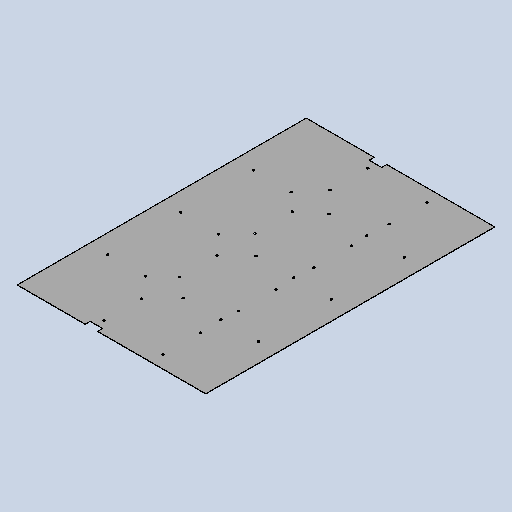
# Autodesk Inventor part: GnG L.3 floor sheet
Saved by Autodesk Inventor 2025.3 (Build 293356030, 356C)
## iProperties
Created: 2025-10-28
Part Number: GnG L.3 floor sheet
Material: Stainless Steel
Document SubType Name: Sheet Metal
Designer: admin
Mass: 82475.6 g
Surface Area: 69006.7 cm^2
Volume: 10309.4 cm^3
Density: 8 g/cm^3
Sheet Metal Rule: AISI304 3mm Die 32
Sheet Metal Width: 1500,000 mm
Sheet Metal Length: 2300,000 mm
Sheet Metal Area: 3450000,000 mm^2
Appearance: Default
Stock Number: L 3
Flat Pattern Width: 150 cm
Flat Pattern Length: 230 cm
Flat Pattern Area: 34500 cm^2
Author: admin
Autodesk Inventor part; units mm, degrees
ref_plane "YZ Plane" through (0, 0, 0) normal (1, 0, 0) x (0, 1, 0)
ref_plane "XZ Plane" through (0, 0, 0) normal (0, 1, 0) x (-1, 0, 0)
ref_plane "XY Plane" through (0, 0, 0) normal (0, 0, 1) x (1, 0, 0)
sketch "Sketch1" plane through (0, 0, 0) normal (0, 0, 1) x (1, 0, 0)
  line L0 (0, 0) -> (-1500, 0)
  line L1 (-1500, 0) -> (-1500, -2300)
  line L2 (-1500, -2300) -> (0, -2300)
  line L3 (0, -2300) -> (0, 0)
  line L4 (0, 0) -> (-40, 0)
  line L5 (-40, 0) -> (-40, -40)
  line L6 (-40, -40) -> (0, -40)
  line L7 (0, -40) -> (0, 0)
  line L8 (0, -2300) -> (-40, -2300)
  line L9 (-40, -2300) -> (-40, -2260)
  line L10 (-40, -2260) -> (0, -2260)
  line L11 (0, -2260) -> (0, -2300)
  line L12 (-1500, 0) -> (-1460, 0)
  line L13 (-1460, 0) -> (-1460, -40)
  line L14 (-1460, -40) -> (-1500, -40)
  line L15 (-1500, -40) -> (-1500, 0)
  line L16 (-1500, -2300) -> (-1460, -2300)
  line L17 (-1460, -2300) -> (-1460, -2260)
  line L18 (-1460, -2260) -> (-1500, -2260)
  line L19 (-1500, -2260) -> (-1500, -2300)
  line L20 (-960, -2300) -> (-860, -2300)
  line L21 (-860, -2300) -> (-860, -2260)
  line L22 (-860, -2260) -> (-960, -2260)
  line L23 (-960, -2260) -> (-960, -2300)
  line L24 (-960, 0) -> (-860, 0)
  line L25 (-860, 0) -> (-860, -40)
  line L26 (-860, -40) -> (-960, -40)
  line L27 (-960, -40) -> (-960, 0)
  point P0 (0, -40)
  point P1 (-40, 0)
  point P2 (0, -2260)
  point P3 (-860, 0)
  dimension "d22" = 1500
  dimension "d23" = 2300
  dimension "d24" = 40
  dimension "d25" = 40
  dimension "d28" = 100
  dimension "d29" = 820
  measures "d22" distance of L2.end L1.end
  measures "d23" distance of L1.end L0.end
  measures "d24" distance of L6.end L5.end
  measures "d25" distance of L5.end L4.end
  measures "d28" distance of L25.end L26.end
  measures "d29" distance between parallel lines of L5 L25
extrude "Plate1" add sketch "Sketch1" along normal blind 3 contours L3 L6 L5 L0 | L5 L6 L3 L10 L9 L2 L21 L22 L23 L17 L18 L1 L14 L13 L0 L27 L26 L25 | L3 L2 L9 L10 | L13 L14 L1 L0 | L18 L17 L2 L1
sketch "Sketch6" plane through (0, 0, 3) normal (0, 0, 1) x (1, 0, 0)
  line L0 (-1395, 0) -> (-1390, 0)
  line L1 (-1375, -2) -> (-1375, 0)
  line L2 (-1375, 0) -> (-1370, 0)
  line L3 (-1370, 0) -> (-1370, -2)
  line L4 (-1370, 0) -> (-1365, 0) construction
  line L5 (-1365, 0) -> (-1363.3887, -1.629)
  arc A0 (-1363.3887, -1.629) -> (-1361.6113, -1.629) centre (-1362.5, -0.75) ccw
  line L6 (-1365, 0) -> (-1360, 0)
  line L7 (-1360, 0) -> (-1355, 0) construction
  line L8 (-1355, -2) -> (-1355, 0)
  line L9 (-1350, -2) -> (-1355, -2)
  line L10 (-1350, 0) -> (-1350, -2)
  line L11 (-1355, 0) -> (-1350, 0)
  line L12 (-1350, -1) -> (-1345, -1) construction
  line L13 (-1361.6113, -1.629) -> (-1360, 0)
  line L14 (-1390, 0) -> (-1390, -2)
  line L15 (-1390, -2) -> (-1395, -2)
  line L16 (-1395, -2) -> (-1395, 0)
  line L17 (-1370, -2) -> (-1375, -2)
  line L18 (-1380, 0) -> (-1380, -2)
  line L19 (-1380, -2) -> (-1385, -2)
  line L20 (-1385, -2) -> (-1385, 0)
  line L21 (-1385, 0) -> (-1380, 0)
  line L22 (-1380, -1) -> (-1375, -1) construction
  line L23 (-1390, -1) -> (-1385, -1) construction
  line L24 (-1345, -2) -> (-1345, 0)
  line L25 (-1340, 0) -> (-1340, -2)
  line L26 (-1340, -2) -> (-1345, -2)
  line L27 (-1345, 0) -> (-1340, 0)
  line L28 (-1340, -1) -> (-1335, -1) construction
  line L29 (-1335, -2) -> (-1335, 0)
  line L30 (-1335, 0) -> (-1330, 0)
  line L31 (-1330, -2) -> (-1335, -2)
  arc A1 (-1402.5, 0) -> (-1397.5, 0) centre (-1400, 0) ccw
  line L32 (-1330, 0) -> (-1330, -2)
  line L33 (-1500, 0) -> (-960, 0) projected
  line L34 (-1500, -2300) -> (-1500, 0) projected
  point P0 (0, 0)
  point P1 (-1362.5, 0)
  dimension "d38" = 5
  dimension "d39" = 2
  dimension "d40" = 1.25
  dimension "d41" = 5
  dimension "d42" = 5
  dimension "d43" = 2
  dimension "d44" = 5
  dimension "d45" = 5
  dimension "d46" = 100
  constraints: 66 end point, 12 parallel, 11 horizontal, 10 equal length, 9 midpoint, 6 perpendicular, 5 collinear, 4 point on circle, 4 point on line, 3 tangent, 2 centre point, 1 vertical alignment
  measures "d38" distance of L14.end L16.start
  measures "d39" distance of L16.start L0.start
  measures "d40" radius of A0
  measures "d41" distance of L5.start L6.end
  measures "d42" distance of L10.end L8.start
  measures "d43" distance of L8.start L7.end
  measures "d44" diameter of A1
  measures "d45" distance of A1.centre L0.start
  measures "d46" distance from line of L34 A1.centre
extrude "Cut1" cut sketch "Sketch6" against normal blind 3 contours L2 L3 L17 L1 | L21 L18 L19 L20 | L0 L14 L15 L16 | A1 L33
sketch "Sketch7" plane through (0, 0, 0) normal (0, 0, -1) x (-1, 0, 0)
  line L0 (1375, 0) -> (1375, -2) construction
  line L1 (1375, -2) -> (1370, -2) construction
  line L2 (1370, -2) -> (1370, 0) construction
  line L3 (960, 0) -> (1370, 0) construction
  line L4 (960, -40) -> (960, 0) construction
  line L5 (860, -40) -> (960, -40) construction
  line L6 (860, 0) -> (860, -40) construction
  line L7 (0, 0) -> (860, 0) construction
  line L8 (0, -2300) -> (0, 0) construction
  line L9 (860, -2300) -> (0, -2300) construction
  line L10 (860, -2260) -> (860, -2300) construction
  line L11 (960, -2260) -> (860, -2260) construction
  line L12 (960, -2300) -> (960, -2260) construction
  line L13 (1500, -2300) -> (960, -2300) construction
  line L14 (1500, 0) -> (1500, -2300) construction
  line L15 (1402.5, 0) -> (1500, 0) construction
  arc A0 (1397.5, 0) -> (1402.5, 0) centre (1400, 0) ccw construction
  line L16 (1395, 0) -> (1397.5, 0) construction
  line L17 (1395, 0) -> (1395, -2) construction
  line L18 (1395, -2) -> (1390, -2) construction
  line L19 (1390, -2) -> (1390, 0) construction
  line L20 (1385, 0) -> (1390, 0) construction
  line L21 (1385, 0) -> (1385, -2) construction
  line L22 (1385, -2) -> (1380, -2) construction
  line L23 (1380, -2) -> (1380, 0) construction
  line L24 (1375, 0) -> (1380, 0) construction
  line L25 (440, 0) -> (440, -2300) construction
  line L26 (910, -2260) -> (910, -40) construction
  line L27 (1500, -570) -> (0, -570) construction
  line L28 (1500, -1150) -> (0, -1150) construction
  line L29 (1500, -1730) -> (0, -1730) construction
  circle A1 centre (440, -2200) radius 7.5
  circle A2 centre (910, -2200) radius 7.5
  circle A3 centre (1350, -570) radius 7.5
  circle A4 centre (1350, -1150) radius 7.5
  circle A5 centre (1350, -1730) radius 7.5
  circle A6 centre (910, -1900) radius 7.5
  circle A7 centre (440, -1900) radius 7.5
  circle A8 centre (910, -1600) radius 7.5
  circle A9 centre (440, -1600) radius 7.5
  circle A10 centre (910, -1300) radius 7.5
  circle A11 centre (440, -1300) radius 7.5
  circle A12 centre (910, -1000) radius 7.5
  circle A13 centre (440, -1000) radius 7.5
  circle A14 centre (910, -700) radius 7.5
  circle A15 centre (440, -700) radius 7.5
  circle A16 centre (910, -400) radius 7.5
  circle A17 centre (440, -400) radius 7.5
  circle A18 centre (910, -100) radius 7.5
  circle A19 centre (440, -100) radius 7.5
  circle A20 centre (910, 200) radius 7.5
  circle A21 centre (440, 200) radius 7.5
  circle A22 centre (910, 500) radius 7.5
  circle A23 centre (440, 500) radius 7.5
  circle A24 centre (910, 800) radius 7.5
  circle A25 centre (440, 800) radius 7.5
  circle A26 centre (1050, -1730) radius 7.5
  circle A27 centre (1050, -570) radius 7.5
  circle A28 centre (1050, -1150) radius 7.5
  circle A29 centre (750, -1730) radius 7.5
  circle A30 centre (750, -570) radius 7.5
  circle A31 centre (750, -1150) radius 7.5
  circle A32 centre (450, -1730) radius 7.5
  circle A33 centre (450, -570) radius 7.5
  circle A34 centre (450, -1150) radius 7.5
  circle A35 centre (150, -1730) radius 7.5
  circle A36 centre (150, -570) radius 7.5
  circle A37 centre (150, -1150) radius 7.5
  circle A38 centre (-150, -1730) radius 7.5
  circle A39 centre (-150, -570) radius 7.5
  circle A40 centre (-150, -1150) radius 7.5
  circle A41 centre (-450, -1730) radius 7.5
  circle A42 centre (-450, -570) radius 7.5
  circle A43 centre (-450, -1150) radius 7.5
  dimension "d49" = 440
  dimension "d50" = 910
  dimension "d51" = 570
  dimension "d52" = 1150
  dimension "d53" = 1730
  dimension "d54" = 15
  dimension "d55" = 100
  dimension "d56" = 150
  dimension "d59" = 300
  dimension "d66" = 300
  constraints: 43 centre point, 11 point on line, 10 end point, 5 perpendicular, 4 equal radius, 4 midpoint, 2 vertical alignment, 1 horizontal, 1 horizontal alignment, 1 vertical, 76 other
  measures "d49" distance between parallel lines of L25 L8
  measures "d50" distance between parallel lines of L26 L8
  measures "d51" distance between parallel lines of L29 L13
  measures "d52" distance between parallel lines of L28 L13
  measures "d53" distance between parallel lines of L27 L13
  measures "d54" diameter of A1
  measures "d55" distance from line of A1.centre L9
  measures "d56" distance from line of A5.centre L14
  measures "d59" distance of A2.centre A6.centre
  measures "d66" distance of A5.centre A26.centre
extrude "Cut2" cut sketch "Sketch7" against normal blind 3
equation "\"d24\" = d25"
equation "\"d40\" = 0.25 * d38"
equation "\"d47\" = Thickness"
equation "\"d71\" = Thickness"
equation "\"d2\" = Thickness"
equation "\"BendReliefWidth\" = Thickness"
equation "\"BendReliefDepth\" = 0.5 * Thickness"
equation "\"CornerReliefSize\" = 4 * Thickness"
equation "\"MinimumRemnant\" = 2 * Thickness"
equation "\"TransitionRadius\" = BendRadius"
equation "\"JacobiRadiusSize\" = BendRadius"
equation "\"GapSize\" = Thickness"
equation "\"Thickness\" = 3"
equation "\"BendRadius\" = 5"
body "Solid1"
